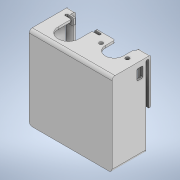
# Autodesk Inventor part: UniversalMount_v1
Saved by Autodesk Inventor 2021 (Build 250183000, 183)
## iProperties
Created: 2021-02-23
Part Number: UniversalMount_v1
Material: Generic
Document SubType Name: Modeling
Designer: allen
Density: 1 g/cm^3
Appearance: Default
Author: allen
Autodesk Inventor part; units mm, degrees
ref_plane "YZ Plane" through (0, 0, 0) normal (1, 0, 0) x (0, 1, 0)
ref_plane "XZ Plane" through (0, 0, 0) normal (0, 1, 0) x (-1, 0, 0)
ref_plane "XY Plane" through (0, 0, 0) normal (0, 0, 1) x (1, 0, 0)
sketch "Sketch1" plane through (0, 0, 0) normal (0, 0, 1) x (1, 0, 0)
  line L0 (-55, -55) -> (55, -55)
  line L1 (55, -55) -> (55, 55)
  line L2 (55, 55) -> (-55, 55)
  line L3 (-55, 55) -> (-55, -55)
  line L4 (-55, -55) -> (55, 55) construction
  line L5 (55, -55) -> (-55, 55) construction
  point P0 (0, 0)
  dimension "d0" = 110
  dimension "d1" = 110
  constraints: 12 end point, 2 midpoint, 2 parallel, 1 horizontal, 1 perpendicular
  measures "d0" distance of L1.end L2.end
  measures "d1" distance of L2.end L0.start
extrude "Extrusion1" add sketch "Sketch1" along normal blind 45
sketch "Sketch8" plane through (-55, 55, 0) normal (0, 1, 0) x (1, 0, 0)
  arc A0 (16.125, -22.8) -> (43.875, -22.8) centre (30, -22.8) ccw
  line L0 (110, 0) -> (0, 0) projected
  line L1 (43.875, -22.8) -> (43.875, 0)
  line L2 (16.125, -22.8) -> (16.125, 0)
  line L3 (43.875, 0) -> (16.125, 0)
  line L4 (0, 0) -> (0, -45) projected
  point P0 (55, 0)
  dimension "d22" = 22.8
  dimension "d23" = 30
  dimension "d24" = 22.8
  dimension "d25" = 22.8
  dimension "d33" = 13.875
  constraints: 6 end point, 2 perpendicular, 2 point on circle, 2 point on line, 1 centre point, 1 collinear
  measures "d22" distance from line of L0 A0.centre
  measures "d23" distance from line of L4 A0.centre
  measures "d24" distance of L2.start L2.end
  measures "d25" distance of L1.start L1.end
  measures "d33" radius of A0
sketch "Sketch9" plane through (0, 0, 0) normal (0, 0, -1) x (-1, 0, 0)
  line L0 (-52, -52) -> (52, -52)
  line L1 (52, -52) -> (52, 52)
  line L2 (52, 52) -> (-52, 52)
  line L3 (-52, 52) -> (-52, -52)
  line L4 (-52, -52) -> (52, 52) construction
  line L5 (52, -52) -> (-52, 52) construction
  line L6 (55, 55) -> (55, -55) projected
  line L7 (-55, 55) -> (55, 55) projected
  point P0 (0, 0)
  dimension "d27" = 3
  dimension "d28" = 3
  constraints: 12 end point, 2 midpoint, 2 parallel, 1 horizontal, 1 perpendicular
  measures "d27" distance between parallel lines of L6 L1
  measures "d28" distance between parallel lines of L2 L7
extrude "Extrusion5" cut sketch "Sketch9" against normal blind 43
extrude "Extrusion6" cut sketch "Sketch8" against normal blind 38
sketch "Sketch10" plane through (0, 0, 0) normal (0, 0, -1) x (-1, 0, 0)
  line L0 (-55, 55) -> (11.125, 55) projected
  line L1 (11.125, 55) -> (-2.875, 55)
  line L2 (-2.875, 55) -> (-2.875, 45)
  line L3 (-2.875, 45) -> (11.125, 45)
  line L4 (11.125, 45) -> (11.125, 55)
  line L5 (38.875, 55) -> (38.875, 52) projected
  line L6 (38.875, 55) -> (54.875, 55)
  line L7 (54.875, 55) -> (54.875, 45)
  line L8 (54.875, 45) -> (38.875, 45)
  line L9 (38.875, 45) -> (38.875, 55)
  circle A0 centre (6.875, 49.5) radius 1.4
  circle A1 centre (43.375, 49.5) radius 1.4
  line L10 (-52, 52) -> (11.125, 52) projected
  line L11 (38.875, 52) -> (52, 52) projected
  point P0 (0, 0)
  dimension "d34" = 10
  dimension "d35" = 14
  dimension "d36" = 2.8
  dimension "d39" = 2.8
  dimension "d42" = 36.5
  dimension "d43" = 4.25
  dimension "d44" = 16
  dimension "d47" = 2.5
  dimension "d48" = 2.5
  constraints: 16 end point, 5 parallel, 2 centre point, 2 horizontal, 2 perpendicular
  measures "d34" distance of L1.end L2.end
  measures "d35" distance of L2.end L3.end
  measures "d36" diameter of A0
  measures "d39" diameter of A1
  measures "d42" distance between centres of A0 A1
  measures "d43" distance from line of L4 A0.centre
  measures "d44" distance of L7.end L8.end
  measures "d47" distance from line of A0.centre L10
  measures "d48" distance from line of L11 A1.centre
extrude "Extrusion7" add sketch "Sketch10" against normal blind 2
sketch "Sketch12" plane through (0, 0, 2) normal (0, 0, 1) x (1, 0, 0)
  line L0 (-1.625, 14.72) -> (-48.375, 14.72)
  line L1 (-48.375, 14.72) -> (-48.375, 55.3239)
  line L2 (-48.375, 55.3239) -> (-1.625, 55.3239)
  line L3 (-1.625, 55.3239) -> (-1.625, 14.72)
  line L4 (-38.875, 55) -> (-38.875, 45) projected
  line L5 (-11.125, 45) -> (-11.125, 55) projected
  point P0 (0, 0)
  dimension "d54" = 9.5
  dimension "d55" = 9.5
  constraints: 8 end point, 2 parallel, 1 horizontal, 1 perpendicular
  measures "d54" distance between parallel lines of L4 L1
  measures "d55" distance between parallel lines of L5 L3
extrude "Extrusion9" cut sketch "Sketch12" along normal blind 3.3
fillet "Fillet4" radius 1.5 10 edges at (-1.625, 53.5, 5.3) (-1.625, 53.5, 2) (-48.375, 53.5, 2) (-48.375, 53.5, 5.3) (-38.875, 53.5, 5.3) (-11.125, 53.5, 5.3) (-11.125, 55, 1) (-38.875, 55, 1) (-38.875, 45, 1) (-11.125, 45, 1)
sketch "Sketch13" plane through (-25, 55, 22.8) normal (0, 1, 0) x (1, 0, 0)
  arc A0 (39, 9.8) -> (63, 9.8) centre (51, 9.8) ccw
  line L0 (63, 9.8) -> (63, 22.8)
  line L1 (-27, 22.8) -> (77, 22.8) projected
  line L2 (39, 9.8) -> (39, 22.8)
  line L3 (51, 9.8) -> (51, -12.8982) construction
  circle A1 centre (68.5, 9.8) radius 2.5
  circle A2 centre (33.5, 9.8) radius 2.5
  line L4 (80, 22.8) -> (80, -22.2) projected
  point P0 (25, 22.8)
  point P1 (-26, 18.2)
  point P2 (96, 18.2)
  dimension "d61" = 13
  dimension "d62" = 13
  dimension "d63" = 12
  dimension "d65" = 17.5
  dimension "d66" = 5
  dimension "d67" = 13
  dimension "d125" = 29
  constraints: 6 end point, 3 centre point, 2 point on circle, 2 vertical, 1 parallel, 1 symmetric about line, 1 tangent, 4 other
  measures "d61" distance of L2.start L2.end
  measures "d62" distance of L0.start L0.end
  measures "d63" radius of A0
  measures "d65" distance from line of L3 A1.centre
  measures "d66" diameter of A1
  measures "d125" distance from line of L4 L3.start
extrude "Extrusion10" cut sketch "Sketch13" against normal blind 5
fillet "Fillet10" radius 4 2 edges at (55, -55, 22.5) (-55, -55, 22.5)
fillet "Fillet12" radius 4 2 edges at (0, 55, 45) (0, 52, 43)
sketch "Sketch22" plane through (-55, -51, 0) normal (-1, 0, 0) x (0, 0, 1)
  line L0 (0, 106) -> (-6.5, 106)
  line L1 (-6.5, 106) -> (-6.5, 46)
  line L2 (-6.5, 46) -> (-4, 46)
  line L3 (-4, 46) -> (-4, 103)
  line L4 (-4, 103) -> (0, 103)
  line L5 (0, 103) -> (0, 106)
  line L6 (0, 97.5) -> (0, 104.5) projected
  point P0 (0, 51)
  dimension "d116" = 6.5
  dimension "d117" = 4
  dimension "d118" = 60
  dimension "d119" = 3
  constraints: 12 end point, 4 perpendicular, 1 collinear, 1 horizontal
  measures "d116" distance of L0.start L0.end
  measures "d117" distance of L3.end L4.end
  measures "d118" distance of L0.end L1.end
  measures "d119" distance of L4.end L0.start
extrude "Extrusion18" add sketch "Sketch22" against normal blind 10
sketch "Sketch23" plane through (55, -51, 0) normal (1, 0, 0) x (0, 0, -1)
  line L0 (6.5, 106) -> (-41, 106) projected
  line L1 (0, 106) -> (6.5, 106)
  line L2 (6.5, 106) -> (6.5, 46) projected
  line L3 (6.5, 106) -> (6.5, 46)
  line L4 (4, 103) -> (4, 46) projected
  line L5 (6.5, 46) -> (4, 46)
  line L6 (0, 103) -> (4, 103) projected
  line L7 (4, 46) -> (4, 103)
  line L8 (4, 103) -> (0, 103)
  line L9 (0, 103) -> (0, 106)
  point P0 (0, 51)
  constraints: 12 end point, 3 collinear, 3 perpendicular
extrude "Extrusion19" add sketch "Sketch23" against normal blind 15
fillet "Fillet14" radius 2 14 edges at (14, 53.5, 0) (2.875, 45, 1) (2.875, 52, 1) (-50, 55, -6.5) (-50, 52, -4) (-50, -5, -6.5) (47.5, -5, -6.5) (47.5, 55, -6.5) (47.5, 52, -4) (40, 53.5, 0) (38, 53.5, 0) (53.5, 52, 0) (-50, 52, 0) (-52, 45, 1)
sketch "Sketch24" plane through (55, -51, 0) normal (1, 0, 0) x (0, 0, -1)
  line L0 (-4, 99) -> (-12, 99)
  line L1 (-12, 99) -> (-12, 85)
  line L2 (-12, 85) -> (-4, 85)
  line L3 (-4, 85) -> (-4, 99)
  line L4 (4.5, 106) -> (-41, 106) projected
  line L5 (0, 0) -> (0, 101) projected
  point P0 (0, 51)
  point P1 (0, 99)
  dimension "d126" = 7
  dimension "d127" = 14
  dimension "d128" = 8
  dimension "d129" = 4
  constraints: 8 end point, 2 parallel, 1 horizontal, 1 perpendicular
  measures "d126" distance between parallel lines of L4 L0
  measures "d127" distance of L2.end L0.start
  measures "d128" distance of L1.end L2.end
  measures "d129" distance between parallel lines of L5 L3
extrude "Extrusion20" cut sketch "Sketch24" against normal blind 15
fillet "Fillet15" radius 1.5 4 edges at (53.5, 48, 12) (53.5, 48, 4) (53.5, 34, 4) (53.5, 34, 12)
sketch "Sketch25" plane through (-51, -55, 0) normal (0, -1, 0) x (1, 0, 0)
  line L0 (23, 33) -> (12, 33)
  line L1 (12, 33) -> (12, 42)
  line L2 (12, 42) -> (23, 42)
  line L3 (23, 42) -> (23, 33)
  line L4 (-1, 0) -> (-1, 43) projected
  line L5 (-1, 43) -> (103, 43) projected
  point P0 (51, 0)
  point P1 (3, 43)
  point P2 (99, 43)
  dimension "d133" = 13
  dimension "d134" = 11
  dimension "d135" = 9
  dimension "d136" = 1
  constraints: 8 end point, 2 parallel, 1 horizontal, 1 perpendicular
  measures "d133" distance between parallel lines of L1 L4
  measures "d134" distance of L0.start L0.end
  measures "d135" distance of L2.end L0.start
  measures "d136" distance between parallel lines of L5 L2
extrude "Extrusion21" cut sketch "Sketch25" against normal blind 10
body "Solid1"
